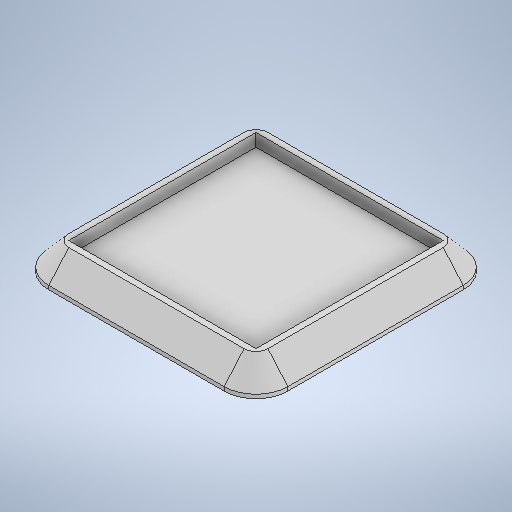
# Autodesk Inventor part: IMU_Base_T-Shirt
Saved by Autodesk Inventor 2025.2 (Build 292293000, 293)
## iProperties
Created: 2024-11-14
Part Number: IMU_Base_T-Shirt
Material: Generic
Document SubType Name: Modeling
Designer: matss
Density: 1 g/cm^3
Appearance: Default
Author: matss
Autodesk Inventor part; units mm, degrees
ref_plane "YZ Plane" through (0, 0, 0) normal (1, 0, 0) x (0, 1, 0)
ref_plane "XZ Plane" through (0, 0, 0) normal (0, 1, 0) x (-1, 0, 0)
ref_plane "XY Plane" through (0, 0, 0) normal (0, 0, 1) x (1, 0, 0)
sketch "Sketch1" plane through (0, 0, 0) normal (0, 1, 0) x (-1, 0, 0)
  line L0 (30, 30) -> (-30, 30)
  line L1 (-30, 30) -> (-30, -30)
  line L2 (-30, -30) -> (30, -30)
  line L3 (30, -30) -> (30, 30)
  point P0 (0, 0)
  point P1 (30, 0)
  point P2 (0, 30)
  dimension "d0" = 60
  dimension "d1" = 60
  constraints: 8 end point, 2 midpoint, 2 parallel, 1 horizontal, 1 horizontal alignment, 1 perpendicular, 1 vertical alignment
  measures "d0" distance of L2.end L0.start
  measures "d1" distance of L0.start L0.end
extrude "Extrusion1" add sketch "Sketch1" along normal blind 0.96
sketch "Sketch2" plane through (0, 0.96, 0) normal (0, 1, 0) x (1, 0, 0)
  line L0 (30, -30) -> (30, 30) projected
  line L1 (30, 30) -> (-30, 30) projected
  line L2 (-30, 30) -> (-30, -30) projected
  line L3 (-30, -30) -> (30, -30) projected
  line L4 (-30, 0) -> (30, 0)
  line L5 (0, -30) -> (0, 30)
  circle A0 centre (-10.5, -10.5) radius 4.25
  circle A1 centre (-10.5, 10.5) radius 4.25
  circle A2 centre (10.5, 10.5) radius 4.25
  circle A3 centre (10.5, -10.5) radius 4.25
  point P0 (0, 0)
  dimension "d13" = 8.5
  dimension "d14" = 21
  dimension "d15" = 21
  constraints: 4 centre point, 4 end point, 4 midpoint, 3 equal radius, 3 other
  measures "d13" diameter of A0
  measures "d14" distance of A3.centre A0.centre
  measures "d15" distance of A1.centre A0.centre
extrude "Extrusion2" add sketch "Sketch2" along normal blind 1.92
sketch "Sketch3" plane through (0, 2.88, 0) normal (0, 1, 0) x (1, 0, 0)
  line L0 (-30, 30) -> (-30, -30) projected
  line L1 (-30, -30) -> (30, -30) projected
  line L2 (30, -30) -> (30, 30) projected
  line L3 (30, 30) -> (-30, 30) projected
  point P0 (0, 0)
extrude "Extrusion3" add sketch "Sketch3" along normal blind 0.64
fillet "Fillet1" radius 8 4 edges at (30, 1.76, 30) (-30, 1.76, 30) (-30, 1.76, -30) (30, 1.76, -30)
ref_plane "Arbeitsebene2" through (27.6569, 3.52, -27.6569) normal (-0.7071068, 0, -0.7071068) x (0, -1, 0)
sketch "Skizze7" plane through (0, 3.52, 0) normal (0, 1, 0) x (1, 0, 0)
  line L0 (-22, -30) -> (22, -30) projected
  arc A0 (22, -30) -> (30, -22) centre (22, -22) ccw projected
  line L1 (30, -22) -> (30, 22) projected
  arc A1 (30, 22) -> (22, 30) centre (22, 22) ccw projected
  line L2 (22, 30) -> (-22, 30) projected
  arc A2 (-22, 30) -> (-30, 22) centre (-22, 22) ccw projected
  line L3 (-30, 22) -> (-30, -22) projected
  arc A3 (-30, -22) -> (-22, -30) centre (-22, -22) ccw projected
  line L4 (22, -30) -> (-22, -30)
  line L5 (-30, -22) -> (-30, 22)
  line L6 (-22, 30) -> (22, 30)
  line L7 (30, 22) -> (30, -22)
  arc A4 (22, -30) -> (30, -22) centre (22, -22) ccw
  arc A5 (-30, -22) -> (-22, -30) centre (-22, -22) ccw
  arc A6 (-22, 30) -> (-30, 22) centre (-22, 22) ccw
  arc A7 (30, 22) -> (22, 30) centre (22, 22) ccw
  point P0 (0, 0)
  constraints: 12 point on circle, 8 end point, 4 centre point, 4 coincident, 3 perpendicular, 1 point on line
extrude "Extrusion4" add sketch "Skizze7" along normal blind 3.2
sketch "Skizze8" plane through (0, 6.72, 0) normal (0, 1, 0) x (1, 0, 0)
  line L0 (23.5, 23.5) -> (-23.5, 23.5)
  line L1 (-23.5, 23.5) -> (-23.5, -23.5)
  line L2 (-23.5, -23.5) -> (23.5, -23.5)
  line L3 (23.5, -23.5) -> (23.5, 23.5)
  line L4 (23.5, 23.5) -> (-23.5, -23.5) construction
  line L5 (-23.5, 23.5) -> (23.5, -23.5) construction
  point P0 (0, 0)
  dimension "d25" = 47
  dimension "d26" = 47
  constraints: 12 end point, 2 midpoint, 2 parallel, 1 horizontal, 1 perpendicular
  measures "d25" distance of L0.end L1.end
  measures "d26" distance of L1.end L2.end
extrude "Extrusion5" cut sketch "Skizze8" against normal blind 3.2
chamfer "Fasen2" distance 5 distance2 5.76 8 edges at (0, 6.72, -30) (-27.6569, 6.72, -27.6569) (-30, 6.72, 0) (-27.6569, 6.72, 27.6569) (0, 6.72, 30) (27.6569, 6.72, 27.6569) (30, 6.72, 0) (27.6569, 6.72, -27.6569) measured on face at (-29.5, 6.72, 0) measured on face at (27.3033, 6.72, 27.3033) measured on face at (-27.3033, 6.72, 27.3033) measured on face at (0, 6.72, 29.5) measured on face at (29.5, 6.72, 0) measured on face at (0, 6.72, -29.5) measured on face at (27.3033, 6.72, -27.3033) measured on face at (-27.3033, 6.72, -27.3033)
body "Solid1"
